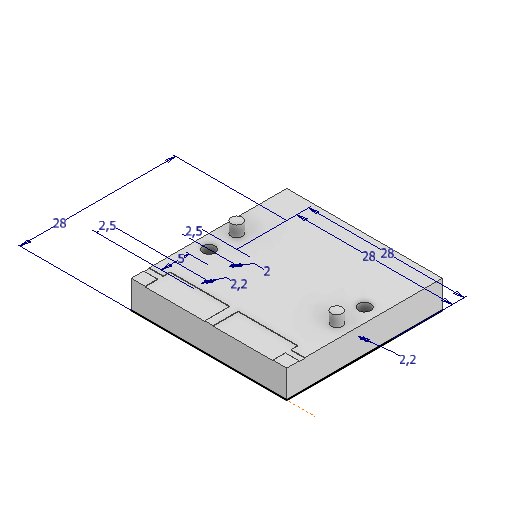
# Autodesk Inventor part: TracciaSotto
Saved by Autodesk Inventor 2025.4 (Build 294407000, 407)
## iProperties
Created: 2026-04-22
Part Number: TracciaSotto
Material: Generic
Document SubType Name: Modeling
Designer: gdira
Density: 1 g/cm^3
Appearance: Default
Author: gdira
Autodesk Inventor part; units mm, degrees
ref_plane "YZ Plane" through (0, 0, 0) normal (1, 0, 0) x (0, 1, 0)
ref_plane "XZ Plane" through (0, 0, 0) normal (0, 1, 0) x (-1, 0, 0)
ref_plane "XY Plane" through (0, 0, 0) normal (0, 0, 1) x (1, 0, 0)
sketch "Sketch1" plane through (0, 0, 0) normal (0, 1, 0) x (-1, 0, 0)
  line L0 (-16.5491, -16.3275) -> (11.4509, -16.3275)
  line L1 (11.4509, 11.6725) -> (-16.5491, 11.6725)
  line L2 (-21.5491, 11.6725) -> (11.4509, 11.6725) construction
  line L3 (-16.5491, 6.6725) -> (-16.5491, -11.3275)
  line L4 (11.4509, 8.6725) -> (11.4509, -11.3275)
  line L5 (11.4509, -7.3275) -> (11.4509, -2.3275)
  line L6 (6.4509, -2.3275) -> (6.4509, -7.3275)
  line L7 (6.4509, -7.3275) -> (11.4509, -7.3275)
  line L8 (11.4509, 2.6725) -> (11.4509, -2.3275)
  line L9 (6.4509, -0.3275) -> (6.4509, 2.6725)
  line L10 (6.4509, 2.6725) -> (11.4509, 2.6725)
  line L11 (11.4509, -7.3275) -> (11.4509, -2.3275)
  line L12 (11.4509, -2.3275) -> (11.4509, 2.6725)
  line L13 (11.4509, 2.6725) -> (11.4509, -2.3275)
  line L14 (11.4509, -2.3275) -> (11.4509, -7.3275)
  line L15 (11.4509, -11.3275) -> (11.4509, -16.3275)
  line L16 (11.4509, 8.6725) -> (11.4509, 11.6725)
  line L17 (-2.5491, -16.3275) -> (-2.5491, 11.6725)
  circle A0 centre (-14.0491, 0.1725) radius 1
  line L18 (-11.5491, 2.6725) -> (-16.5491, 2.6725)
  line L19 (-16.5491, 2.6725) -> (-16.5491, -2.3275)
  line L20 (-16.5491, -2.3275) -> (-16.5491, 2.6725)
  line L21 (-16.5491, 2.6725) -> (-16.5491, -2.3275)
  line L22 (-11.5491, -0.3275) -> (-11.5491, 2.6725)
  circle A1 centre (-14.0491, -4.8275) radius 1.1
  line L23 (-16.5491, -7.3275) -> (-16.5491, -2.3275)
  line L24 (-16.5491, -7.3275) -> (-16.5491, -2.3275)
  line L25 (-16.5491, -2.3275) -> (-16.5491, -7.3275)
  line L26 (-11.5491, -2.3275) -> (-11.5491, -7.3275)
  line L27 (-11.5491, -7.3275) -> (-16.5491, -7.3275)
  line L28 (-16.5491, -11.3275) -> (-16.5491, -16.3275)
  line L29 (-16.5491, 8.6725) -> (-16.5491, -11.3275)
  line L30 (-16.5491, 11.6725) -> (-16.5491, -16.3275)
  line L31 (8.9509, -4.8275) -> (11.4509, -4.8275)
  line L32 (8.9509, 0.1725) -> (11.4509, 0.1725)
  circle A2 centre (8.9509, -4.8275) radius 1
  circle A3 centre (8.9509, 0.1725) radius 1.1
  point P0 (0, 0)
  point P1 (8.9509, -7.3275)
  point P2 (8.9509, 2.6725)
  point P3 (-14.0491, 2.6725)
  point P4 (-14.0491, -7.3275)
  point P5 (11.4509, 2.6725)
  point P6 (-16.5491, 2.6725)
  point P7 (11.4509, -7.3275)
  dimension "d0" = 5
  dimension "d1" = 2.5
  dimension "d2" = 2.5
  dimension "d3" = 2
  dimension "d4" = 2.2
  dimension "d5" = 2.2
  dimension "d6" = 28
  dimension "d7" = 28
  dimension "d14" = 28
  constraints: 66 end point, 14 symmetric about line, 5 midpoint, 4 centre point, 3 perpendicular, 3 point on line, 2 coincident, 1 horizontal, 1 parallel
  measures "d0" distance of L8.start L8.end
  measures "d1" distance of point (8.951, -7.327) L31.start
  measures "d2" distance of point (8.951, 2.673) L32.start
  measures "d3" diameter of A2
  measures "d4" diameter of A3
  measures "d5" diameter of A1
  measures "d6" distance between parallel lines of L23 L5
  measures "d7" distance between parallel lines of L1 L0
  measures "d14" distance of L0.start L15.end
extrude "Extrusion1" add sketch "Sketch1" along normal blind 5
extrude "Extrusion2" add sketch "Sketch1" along normal blind 7 contours A2 | A0
extrude "Extrusion3" add sketch "Sketch1" along normal blind 2.8 contours A3 | A1
sketch "Sketch2" plane through (0, 5, 0) normal (0, 1, 0) x (1, 0, 0)
  line L0 (-11.4509, -11.6725) -> (16.5491, -11.6725) projected
  line L1 (2.5491, -11.6725) -> (14.0491, -11.6725)
  line L2 (14.0491, -11.6725) -> (14.0491, -7.1725)
  line L3 (14.0491, -7.1725) -> (-8.9509, -7.1725)
  line L4 (-8.9509, -7.1725) -> (-8.9509, -11.6725)
  line L5 (2.5491, -11.6725) -> (3.2991, -11.6725)
  line L6 (3.2991, -11.6725) -> (1.7991, -11.6725)
  line L7 (1.7991, -11.6725) -> (1.7991, -7.1725)
  line L8 (1.7991, -7.1725) -> (3.2991, -7.1725)
  line L9 (3.2991, -7.1725) -> (3.2991, -11.6725)
  line L10 (3.2991, -11.6725) -> (1.7991, -11.6725)
  line L11 (-11.4509, 16.3275) -> (-11.4509, -11.6725) projected
  line L12 (-8.9509, -9.4225) -> (-11.4509, -9.4225)
  line L13 (-11.4509, -9.4225) -> (-11.4509, -8.4225)
  line L14 (-11.4509, -8.4225) -> (-8.9509, -8.4225)
  line L15 (-8.9509, -8.4225) -> (-8.9509, -9.4225)
  line L16 (14.0491, -9.4225) -> (14.0491, -8.4225)
  line L17 (14.0491, -8.4225) -> (16.5491, -8.4225)
  line L18 (16.5491, -8.4225) -> (16.5491, -9.4225)
  line L19 (16.5491, -9.4225) -> (14.0491, -9.4225)
  point P0 (0, 0)
  dimension "d15" = 11.5
  dimension "d16" = 4.5
  dimension "d17" = 23
  dimension "d18" = 0.75
  dimension "d19" = 1.5
  dimension "d20" = 1
  constraints: 36 end point, 8 point on line, 7 perpendicular, 6 parallel, 3 midpoint, 1 horizontal
  measures "d15" distance of L1.start L1.end
  measures "d16" distance of L1.end L2.end
  measures "d17" distance of L2.end L3.end
  measures "d18" distance of L1.start L5.end
  measures "d19" distance of L5.end L6.end
  measures "d20" distance of L12.end L13.end
extrude "Extrusion4" cut sketch "Sketch2" against normal blind 0.1 contours L4 L3 L7 L0 | L11 L14 L4 L12 | L9 L3 L2 L0 | L2 L17 L18 L19
body "Solid1"
